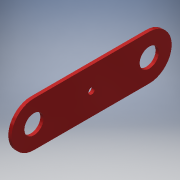
# Autodesk Inventor part: Swing Arm
Saved by Autodesk Inventor 2017 (Build 210142000, 142)
## iProperties
Created: 2017-01-14
Part Number: Swing Arm
Material: Generic
Document SubType Name: Modeling
Designer: Ben
Density: 1 g/cm^3
Appearance: Light Red
Author: Ben
Autodesk Inventor part; units mm, degrees
ref_plane "YZ Plane" through (0, 0, 0) normal (1, 0, 0) x (0, 1, 0)
ref_plane "XZ Plane" through (0, 0, 0) normal (0, 1, 0) x (-1, 0, 0)
ref_plane "XY Plane" through (0, 0, 0) normal (0, 0, 1) x (1, 0, 0)
sketch "Sketch1" plane through (0, 0, 0) normal (1, 0, 0) x (0, 1, 0)
  circle A0 centre (0, 0) radius 9.525
  circle A1 centre (0, -114.3) radius 9.525
  line L0 (0, -114.3) -> (0, 0) construction
  circle A2 centre (0, -57.15) radius 3.175
  arc A3 (22.225, 0) -> (-22.225, 0) centre (0, 0) ccw
  arc A4 (-22.225, -114.3) -> (22.225, -114.3) centre (0, -114.3) ccw
  line L1 (22.225, 0) -> (22.225, -114.3)
  line L2 (0, -57.15) -> (-50.8, -57.15) construction
  circle A5 centre (-50.8, -57.15) radius 3.175
  arc A6 (-50.8, -44.45) -> (-50.8, -69.85) centre (-50.8, -57.15) ccw
  line L3 (-22.225, 0) -> (-22.225, -31.75)
  line L4 (-22.225, -114.3) -> (-22.225, -82.55)
  line L5 (-50.8, -44.45) -> (-34.925, -44.45)
  line L6 (-50.8, -69.85) -> (-34.925, -69.85)
  arc A7 (-34.925, -44.45) -> (-22.225, -31.75) centre (-34.925, -31.75) ccw
  arc A8 (-22.225, -82.55) -> (-34.925, -69.85) centre (-34.925, -82.55) ccw
  dimension "d1" = 19.05
  dimension "d3" = 114.3
  dimension "d4" = 6.35
  dimension "d5" = 44.45
  dimension "d16" = 50.8
  dimension "d17" = 6.35
  dimension "d18" = 25.4
  constraints: 14 end point, 10 point on circle, 9 centre point, 9 tangent, 5 coincident, 4 equal radius, 4 vertical, 3 horizontal, 1 midpoint
  measures "d1" diameter of A0
  measures "d3" distance of point (0, 0) L0.start
  measures "d4" diameter of A2
  measures "d5" diameter of A3
  measures "d16" distance of L2.start L2.end
  measures "d17" diameter of A5
  measures "d18" diameter of A6
extrude "Extrusion1" add sketch "Sketch1" along normal blind 3.175
body "Solid1"
